Autodesk Fusion 360 part; units mm, degrees
(part 6 of 8)
  line L127 (16.3165, -98.3227) -> (16.3216, -98.4252)
  spline S1733 degree 3 poles (16.3216, -98.4252) (16.3211, -98.483) (16.3393, -98.5285) (16.3548, -98.5317) knots 0 0 0 0 1 1 1 1
  spline S1734 degree 3 poles (16.3548, -98.5317) (16.3752, -98.5342) (16.3906, -98.8238) (16.3886, -99.1759) knots 0 0 0 0 1 1 1 1
  spline S1735 degree 3 poles (16.3886, -99.1759) (16.3893, -99.7137) (16.3719, -99.8792) (16.278, -100.2401) knots 0 0 0 0 1 1 1 1
  spline S1736 degree 3 poles (16.278, -100.2401) (16.2147, -100.4816) (16.1437, -100.6813) (16.1109, -100.7004) knots 0 0 0 0 1 1 1 1
  spline S1737 degree 3 poles (16.1109, -100.7004) (16.0808, -100.7217) (16.069, -100.7483) (16.0801, -100.7569) knots 0 0 0 0 1 1 1 1
  spline S1738 degree 3 poles (16.0801, -100.7569) (16.094, -100.7678) (15.9885, -100.8913) (15.8475, -101.0318) knots 0 0 0 0 1 1 1 1
  spline S1739 degree 3 poles (15.8475, -101.0318) (15.7042, -101.1751) (15.5774, -101.3088) (15.5594, -101.326) knots 0 0 0 0 1 1 1 1
  spline S1740 degree 3 poles (15.5594, -101.326) (15.5442, -101.3455) (15.5244, -101.3479) (15.5198, -101.3309) knots 0 0 0 0 1 1 1 1
  spline S1741 degree 3 poles (15.5198, -101.3309) (15.5124, -101.3117) (15.4904, -101.3169) (15.473, -101.3392) knots 0 0 0 0 1 1 1 1
  spline S1742 degree 3 poles (15.473, -101.3392) (15.4448, -101.3753) (15.4503, -101.3796) (15.5098, -101.3724) knots 0 0 0 0 1 1 1 1
  spline S1743 degree 3 poles (15.5098, -101.3724) (15.5472, -101.3703) (15.7087, -101.2323) (15.8901, -101.0517) knots 0 0 0 0 1 1 1 1
  line L128 (15.8901, -101.0517) -> (16.2039, -100.7417)
  line L129 (16.2039, -100.7417) -> (16.3228, -100.2974)
  spline S1744 degree 3 poles (16.3228, -100.2974) (16.4479, -99.8221) (16.4656, -99.7822) (16.538, -99.7985) knots 0 0 0 0 1 1 1 1
  spline S1745 degree 3 poles (16.538, -99.7985) (16.5618, -99.8081) (16.555, -99.7939) (16.5195, -99.7706) knots 0 0 0 0 1 1 1 1
  spline S1746 degree 3 poles (16.5195, -99.7706) (16.454, -99.7284) (16.4546, -99.6931) (16.4526, -96.2577) knots 0 0 0 0 1 1 1 1
  spline S1747 degree 3 poles (16.4526, -96.2577) (16.4536, -95.6318) (16.4543, -95.0235) (16.4558, -94.9128) knots 0 0 0 0 1 1 1 1
  spline S1748 degree 3 poles (16.4558, -94.9128) (16.4567, -94.797) (16.4542, -94.2042) (16.4543, -93.591) knots 0 0 0 0 1 1 1 1
  spline S1749 degree 3 poles (16.4543, -93.591) (16.4524, -89.2558) (16.4467, -89.7215) (16.5046, -89.7219) knots 0 0 0 0 1 1 1 1
  spline S1750 degree 3 poles (16.5046, -89.7219) (16.525, -89.7245) (16.6036, -89.7098) (16.6773, -89.6957) knots 0 0 0 0 1 1 1 1
  spline S1751 degree 3 poles (16.6773, -89.6957) (16.7998, -89.6706) (16.7971, -89.6684) (16.6352, -89.6808) knots 0 0 0 0 1 1 1 1
  line L130 (16.6352, -89.6808) -> (16.4585, -89.6949)
  line L131 (16.4585, -89.6949) -> (16.4072, -89.5429)
  spline S1752 degree 3 poles (16.4072, -89.5429) (16.3814, -89.4556) (16.3356, -89.3079) (16.308, -89.2057) knots 0 0 0 0 1 1 1 1
  spline S1753 degree 3 poles (16.308, -89.2057) (16.281, -89.1085) (16.2542, -89.0339) (16.2455, -89.045) knots 0 0 0 0 1 1 1 1
  spline S1754 degree 3 poles (16.2455, -89.045) (16.2368, -89.0561) (16.2298, -89.0193) (16.2274, -88.9593) knots 0 0 0 0 1 1 1 1
  line L132 (16.2274, -88.9593) -> (16.2274, -88.8562)
  line L133 (16.2274, -88.8562) -> (16.1628, -88.9446)
  spline S1755 degree 3 poles (16.1628, -88.9446) (16.1222, -89.0023) (16.1096, -89.0642) (16.1256, -89.1125) knots 0 0 0 0 1 1 1 1
  spline S1756 degree 3 poles (16.3207, -89.3499) (16.3449, -89.445) (16.358, -89.5313) (16.3515, -89.5397) knots 0 0 0 0 1 1 1 1
  spline S1757 degree 3 poles (16.3515, -89.5397) (16.3471, -89.5452) (16.3232, -89.4728) (16.2989, -89.3777) knots 0 0 0 0 1 1 1 1
  spline S1758 degree 3 poles (16.2989, -89.3777) (16.2747, -89.2827) (16.2616, -89.1963) (16.2681, -89.188) knots 0 0 0 0 1 1 1 1
  spline S1759 degree 3 poles (16.2681, -89.188) (16.2724, -89.1824) (16.2964, -89.2549) (16.3207, -89.3499) knots 0 0 0 0 1 1 1 1
  spline S1760 degree 3 poles (16.3839, -89.5784) (16.3895, -89.5828) (16.3943, -89.6224) (16.3942, -89.6626) knots 0 0 0 0 1 1 1 1
  spline S1761 degree 3 poles (16.3942, -89.6626) (16.3956, -89.7353) (16.3907, -89.7359) (16.3744, -89.665) knots 0 0 0 0 1 1 1 1
  spline S1762 degree 3 poles (16.3744, -89.665) (16.3582, -89.5941) (16.3617, -89.561) (16.3839, -89.5784) knots 0 0 0 0 1 1 1 1
  spline S1763 degree 3 poles (16.3869, -97.9748) (16.3958, -98.0265) (16.3926, -98.0822) (16.3795, -98.0989) knots 0 0 0 0 1 1 1 1
  spline S1764 degree 3 poles (16.3795, -98.0989) (16.3637, -98.1134) (16.3517, -98.0771) (16.3522, -98.0193) knots 0 0 0 0 1 1 1 1
  spline S1765 degree 3 poles (16.3522, -98.0193) (16.3451, -97.8794) (16.3646, -97.8544) (16.3869, -97.9748) knots 0 0 0 0 1 1 1 1
  spline S1766 degree 3 poles (6.4751, -101.6422) (6.4707, -101.688) (6.4876, -101.7236) (6.5074, -101.7212) knots 0 0 0 0 1 1 1 1
  spline S1767 degree 3 poles (6.5074, -101.7212) (6.5272, -101.7188) (6.5375, -101.6999) (6.5295, -101.6758) knots 0 0 0 0 1 1 1 1
  spline S1768 degree 3 poles (6.5295, -101.6758) (6.5215, -101.6516) (6.5238, -101.6086) (6.5328, -101.5799) knots 0 0 0 0 1 1 1 1
  spline S1769 degree 3 poles (6.5328, -101.5799) (6.5424, -101.5561) (6.535, -101.5369) (6.5137, -101.547) knots 0 0 0 0 1 1 1 1
  spline S1770 degree 3 poles (6.5137, -101.547) (6.4917, -101.5522) (6.4746, -101.5971) (6.4751, -101.6422) knots 0 0 0 0 1 1 1 1
  spline S1771 degree 3 poles (16.7866, -88.5186) (16.8252, -88.5667) (16.8384, -88.5726) (16.8336, -88.533) knots 0 0 0 0 1 1 1 1
  spline S1772 degree 3 poles (16.8336, -88.533) (16.8305, -88.5082) (16.8065, -88.476) (16.7827, -88.4663) knots 0 0 0 0 1 1 1 1
  spline S1773 degree 3 poles (16.7827, -88.4663) (16.7539, -88.4573) (16.7591, -88.4793) (16.7866, -88.5186) knots 0 0 0 0 1 1 1 1
  spline S1774 degree 3 poles (6.7487, -102.0083) (6.7647, -102.0566) (6.7792, -102.0724) (6.7833, -102.0442) knots 0 0 0 0 1 1 1 1
  spline S1775 degree 3 poles (6.7833, -102.0442) (6.7852, -102.0189) (6.8218, -101.9892) (6.8636, -101.9816) knots 0 0 0 0 1 1 1 1
  spline S1776 degree 3 poles (6.8636, -101.9816) (6.9268, -101.9638) (6.9268, -101.9638) (6.8711, -101.9606) knots 0 0 0 0 1 1 1 1
  spline S1777 degree 3 poles (6.8711, -101.9606) (6.8358, -101.9599) (6.7845, -101.9511) (6.7606, -101.9414) knots 0 0 0 0 1 1 1 1
  spline S1778 degree 3 poles (6.7606, -101.9414) (6.7319, -101.9324) (6.7272, -101.9556) (6.7487, -102.0083) knots 0 0 0 0 1 1 1 1
  spline S1779 degree 3 poles (8.4157, -99.7829) (8.4296, -99.7938) (8.4739, -99.8059) (8.507, -99.8094) knots 0 0 0 0 1 1 1 1
  spline S1780 degree 3 poles (8.507, -99.8094) (8.5401, -99.8129) (8.5565, -99.8033) (8.5426, -99.7925) knots 0 0 0 0 1 1 1 1
  spline S1781 degree 3 poles (8.5426, -99.7925) (8.5259, -99.7794) (8.4845, -99.7695) (8.4514, -99.766) knots 0 0 0 0 1 1 1 1
  spline S1782 degree 3 poles (8.4514, -99.766) (8.4183, -99.7625) (8.3991, -99.7699) (8.4157, -99.7829) knots 0 0 0 0 1 1 1 1
  spline S1783 degree 3 poles (16.9973, -89.2116) (17.0136, -89.2824) (17.0185, -89.2818) (17.0171, -89.2091) knots 0 0 0 0 1 1 1 1
  spline S1784 degree 3 poles (17.0171, -89.2091) (17.0172, -89.1689) (17.0124, -89.1293) (17.0068, -89.1249) knots 0 0 0 0 1 1 1 1
  spline S1785 degree 3 poles (17.0068, -89.1249) (16.9846, -89.1076) (16.9811, -89.1407) (16.9973, -89.2116) knots 0 0 0 0 1 1 1 1
  spline S1786 degree 3 poles (8.7033, -99.8733) (8.7172, -99.8841) (8.7614, -99.8963) (8.7945, -99.8998) knots 0 0 0 0 1 1 1 1
  spline S1787 degree 3 poles (8.7945, -99.8998) (8.8276, -99.9032) (8.844, -99.8937) (8.8301, -99.8828) knots 0 0 0 0 1 1 1 1
  spline S1788 degree 3 poles (8.8301, -99.8828) (8.8134, -99.8698) (8.772, -99.8598) (8.7389, -99.8563) knots 0 0 0 0 1 1 1 1
  spline S1789 degree 3 poles (8.7389, -99.8563) (8.7058, -99.8529) (8.6866, -99.8602) (8.7033, -99.8733) knots 0 0 0 0 1 1 1 1
  spline S1790 degree 3 poles (11.2338, -96.6572) (11.2477, -96.6681) (11.2824, -96.6638) (11.3103, -96.6453) knots 0 0 0 0 1 1 1 1
  spline S1791 degree 3 poles (11.3103, -96.6453) (11.3546, -96.6173) (11.354, -96.6123) (11.294, -96.6147) knots 0 0 0 0 1 1 1 1
  spline S1792 degree 3 poles (11.294, -96.6147) (11.2163, -96.6167) (11.1977, -96.629) (11.2338, -96.6572) knots 0 0 0 0 1 1 1 1
  spline S1793 degree 3 poles (17.0434, -89.3818) (17.0596, -89.4527) (17.0646, -89.4521) (17.0632, -89.3794) knots 0 0 0 0 1 1 1 1
  spline S1794 degree 3 poles (17.0632, -89.3794) (17.0633, -89.3392) (17.0584, -89.2996) (17.0528, -89.2952) knots 0 0 0 0 1 1 1 1
  spline S1795 degree 3 poles (17.0528, -89.2952) (17.0306, -89.2778) (17.0271, -89.3109) (17.0434, -89.3818) knots 0 0 0 0 1 1 1 1
  spline S1796 degree 3 poles (15.3767, -91.5895) (15.3841, -91.6087) (15.4023, -91.614) (15.4132, -91.6001) knots 0 0 0 0 1 1 1 1
  spline S1797 degree 3 poles (15.4132, -91.6001) (15.4262, -91.5834) (15.4232, -91.5587) (15.4093, -91.5478) knots 0 0 0 0 1 1 1 1
  spline S1798 degree 3 poles (15.4093, -91.5478) (15.3926, -91.5348) (15.3772, -91.5317) (15.3728, -91.5372) knots 0 0 0 0 1 1 1 1
  spline S1799 degree 3 poles (15.3728, -91.5372) (15.3663, -91.5456) (15.3666, -91.5682) (15.3767, -91.5895) knots 0 0 0 0 1 1 1 1
  spline S1800 degree 3 poles (17.0851, -89.5577) (17.0917, -89.6121) (17.0843, -89.6332) (17.062, -89.6158) knots 0 0 0 0 1 1 1 1
  spline S1801 degree 3 poles (17.062, -89.6158) (17.0426, -89.6006) (17.0178, -89.6036) (17.0026, -89.6231) knots 0 0 0 0 1 1 1 1
  spline S1802 degree 3 poles (17.0026, -89.6231) (16.9831, -89.6481) (16.9914, -89.6546) (17.036, -89.6491) knots 0 0 0 0 1 1 1 1
  spline S1803 degree 3 poles (17.036, -89.6491) (17.0805, -89.6437) (17.0978, -89.6617) (17.1141, -89.7325) knots 0 0 0 0 1 1 1 1
  spline S1804 degree 3 poles (17.1141, -89.7325) (17.1257, -89.7864) (17.1258, -89.7462) (17.1214, -89.6487) knots 0 0 0 0 1 1 1 1
  spline S1805 degree 3 poles (17.1214, -89.6487) (17.112, -89.5518) (17.1017, -89.4677) (17.0961, -89.4633) knots 0 0 0 0 1 1 1 1
  spline S1806 degree 3 poles (17.0961, -89.4633) (17.0794, -89.4503) (17.0775, -89.4757) (17.0851, -89.5577) knots 0 0 0 0 1 1 1 1
  spline S1807 degree 3 poles (9.0301, -99.9764) (9.0616, -99.9876) (9.099, -100.0257) (9.1088, -100.0648) knots 0 0 0 0 1 1 1 1
  spline S1808 degree 3 poles (9.1088, -100.0648) (9.1232, -100.1208) (9.126, -100.123) (9.1221, -100.0707) knots 0 0 0 0 1 1 1 1
  spline S1809 degree 3 poles (9.1221, -100.0707) (9.121, -100.0205) (9.1498, -99.9893) (9.2638, -99.9351) knots 0 0 0 0 1 1 1 1
  spline S1810 degree 3 poles (9.2638, -99.9351) (9.3416, -99.8929) (9.3722, -99.8766) (9.3289, -99.892) knots 0 0 0 0 1 1 1 1
  spline S1811 degree 3 poles (9.3289, -99.892) (9.2877, -99.9046) (9.1871, -99.9245) (9.1106, -99.9364) knots 0 0 0 0 1 1 1 1
  spline S1812 degree 3 poles (9.1106, -99.9364) (9.0243, -99.9495) (8.9936, -99.9658) (9.0301, -99.9764) knots 0 0 0 0 1 1 1 1
  spline S1813 degree 3 poles (11.9407, -96.5604) (12.1041, -96.5403) (12.2422, -96.5184) (12.2465, -96.5128) knots 0 0 0 0 1 1 1 1
  spline S1814 degree 3 poles (12.2465, -96.5128) (12.253, -96.5045) (12.1259, -96.5125) (11.9625, -96.5326) knots 0 0 0 0 1 1 1 1
  spline S1815 degree 3 poles (11.9625, -96.5326) (11.799, -96.5527) (11.661, -96.5746) (11.6567, -96.5802) knots 0 0 0 0 1 1 1 1
  spline S1816 degree 3 poles (11.6567, -96.5802) (11.6501, -96.5885) (11.7773, -96.5805) (11.9407, -96.5604) knots 0 0 0 0 1 1 1 1
  line L134 (17.1133, -89.9513) -> (17.136, -90.0541)
  line L135 (17.136, -90.0541) -> (17.1331, -89.9489)
  spline S1817 degree 3 poles (17.1331, -89.9489) (17.1287, -89.8514) (17.1195, -89.8173) (17.1021, -89.8396) knots 0 0 0 0 1 1 1 1
  spline S1818 degree 3 poles (17.1021, -89.8396) (17.0977, -89.8451) (17.1038, -89.8947) (17.1133, -89.9513) knots 0 0 0 0 1 1 1 1
  spline S1819 degree 3 poles (7.9987, -101.606) (8.0126, -101.6168) (8.0374, -101.6138) (8.0504, -101.5971) knots 0 0 0 0 1 1 1 1
  spline S1820 degree 3 poles (8.0504, -101.5971) (8.0613, -101.5832) (8.0517, -101.5668) (8.0313, -101.5643) knots 0 0 0 0 1 1 1 1
  spline S1821 degree 3 poles (8.0313, -101.5643) (8.0081, -101.5596) (7.9861, -101.5648) (7.9796, -101.5731) knots 0 0 0 0 1 1 1 1
  spline S1822 degree 3 poles (7.9796, -101.5731) (7.9752, -101.5787) (7.982, -101.5929) (7.9987, -101.606) knots 0 0 0 0 1 1 1 1
  spline S1823 degree 3 poles (7.3497, -102.6658) (7.4478, -102.6663) (7.5348, -102.6582) (7.5413, -102.6498) knots 0 0 0 0 1 1 1 1
  spline S1824 degree 3 poles (7.5413, -102.6498) (7.5456, -102.6443) (7.4695, -102.6385) (7.3714, -102.638) knots 0 0 0 0 1 1 1 1
  spline S1825 degree 3 poles (7.3714, -102.638) (7.2734, -102.6375) (7.1864, -102.6457) (7.1799, -102.654) knots 0 0 0 0 1 1 1 1
  spline S1826 degree 3 poles (7.1799, -102.654) (7.1755, -102.6596) (7.2516, -102.6653) (7.3497, -102.6658) knots 0 0 0 0 1 1 1 1
  line L136 (9.1141, -100.333) -> (9.1398, -100.4606)
  line L137 (9.1398, -100.4606) -> (9.1339, -100.3306)
  spline S1827 degree 3 poles (9.1339, -100.3306) (9.1276, -100.2585) (9.1203, -100.1991) (9.1147, -100.1947) knots 0 0 0 0 1 1 1 1
  spline S1828 degree 3 poles (9.1147, -100.1947) (9.0925, -100.1773) (9.0946, -100.2148) (9.1141, -100.333) knots 0 0 0 0 1 1 1 1
  spline S1829 degree 3 poles (9.4989, -99.8233) (9.5072, -99.8299) (9.5462, -99.82) (9.5868, -99.8025) knots 0 0 0 0 1 1 1 1
  spline S1830 degree 3 poles (9.5868, -99.8025) (9.6274, -99.7849) (9.6525, -99.7643) (9.6469, -99.7599) knots 0 0 0 0 1 1 1 1
  spline S1831 degree 3 poles (9.6469, -99.7599) (9.6386, -99.7534) (9.5996, -99.7632) (9.559, -99.7808) knots 0 0 0 0 1 1 1 1
  spline S1832 degree 3 poles (9.559, -99.7808) (9.5184, -99.7983) (9.4933, -99.819) (9.4989, -99.8233) knots 0 0 0 0 1 1 1 1
  spline S1833 degree 3 poles (17.1128, -90.1524) (17.1291, -90.2233) (17.134, -90.2227) (17.1327, -90.15) knots 0 0 0 0 1 1 1 1
  spline S1834 degree 3 poles (17.1327, -90.15) (17.1327, -90.1098) (17.1279, -90.0701) (17.1223, -90.0658) knots 0 0 0 0 1 1 1 1
  spline S1835 degree 3 poles (17.1223, -90.0658) (17.1001, -90.0484) (17.0966, -90.0815) (17.1128, -90.1524) knots 0 0 0 0 1 1 1 1
  line L138 (9.1228, -100.6084) -> (9.1485, -100.7359)
  line L139 (9.1485, -100.7359) -> (9.1426, -100.606)
  spline S1836 degree 3 poles (9.1426, -100.606) (9.1363, -100.5339) (9.129, -100.4745) (9.1234, -100.4701) knots 0 0 0 0 1 1 1 1
  spline S1837 degree 3 poles (9.1234, -100.4701) (9.1012, -100.4527) (9.1032, -100.4902) (9.1228, -100.6084) knots 0 0 0 0 1 1 1 1
  line L140 (17.1124, -90.3535) -> (17.1351, -90.4563)
  line L141 (17.1351, -90.4563) -> (17.1322, -90.3511)
  spline S1838 degree 3 poles (17.1322, -90.3511) (17.1278, -90.2536) (17.1186, -90.2196) (17.1012, -90.2418) knots 0 0 0 0 1 1 1 1
  spline S1839 degree 3 poles (17.1012, -90.2418) (17.0969, -90.2474) (17.1029, -90.2969) (17.1124, -90.3535) knots 0 0 0 0 1 1 1 1
  spline S1840 degree 3 poles (7.752, -102.6667) (7.85, -102.6672) (7.937, -102.6591) (7.9435, -102.6507) knots 0 0 0 0 1 1 1 1
  spline S1841 degree 3 poles (7.9435, -102.6507) (7.9479, -102.6452) (7.8718, -102.6394) (7.7737, -102.6389) knots 0 0 0 0 1 1 1 1
  spline S1842 degree 3 poles (7.7737, -102.6389) (7.6756, -102.6384) (7.5886, -102.6465) (7.5821, -102.6549) knots 0 0 0 0 1 1 1 1
  spline S1843 degree 3 poles (7.5821, -102.6549) (7.5778, -102.6604) (7.6539, -102.6662) (7.752, -102.6667) knots 0 0 0 0 1 1 1 1
  spline S1844 degree 3 poles (17.112, -90.5546) (17.1282, -90.6255) (17.1332, -90.6249) (17.1318, -90.5522) knots 0 0 0 0 1 1 1 1
  spline S1845 degree 3 poles (17.1318, -90.5522) (17.1304, -90.4795) (17.119, -90.4482) (17.1016, -90.4705) knots 0 0 0 0 1 1 1 1
  spline S1846 degree 3 poles (17.1016, -90.4705) (17.0973, -90.476) (17.1022, -90.5156) (17.112, -90.5546) knots 0 0 0 0 1 1 1 1
  spline S1847 degree 3 poles (7.2792, -103.2374) (7.2847, -103.2418) (7.3243, -103.2369) (7.3655, -103.2243) knots 0 0 0 0 1 1 1 1
  spline S1848 degree 3 poles (7.3655, -103.2243) (7.4342, -103.2109) (7.4336, -103.2059) (7.3609, -103.2073) knots 0 0 0 0 1 1 1 1
  spline S1849 degree 3 poles (7.3609, -103.2073) (7.2882, -103.2087) (7.2569, -103.2201) (7.2792, -103.2374) knots 0 0 0 0 1 1 1 1
  line L142 (17.1115, -90.7557) -> (17.1342, -90.8585)
  line L143 (17.1342, -90.8585) -> (17.1313, -90.7533)
  spline S1850 degree 3 poles (17.1313, -90.7533) (17.1269, -90.6558) (17.1177, -90.6218) (17.1003, -90.644) knots 0 0 0 0 1 1 1 1
  spline S1851 degree 3 poles (17.1003, -90.644) (17.096, -90.6496) (17.1021, -90.6991) (17.1115, -90.7557) knots 0 0 0 0 1 1 1 1
  spline S1852 degree 3 poles (13.8781, -94.9402) (13.8854, -94.9594) (13.9037, -94.9647) (13.9145, -94.9508) knots 0 0 0 0 1 1 1 1
  spline S1853 degree 3 poles (13.9145, -94.9508) (13.9276, -94.9342) (13.9245, -94.9094) (13.9106, -94.8985) knots 0 0 0 0 1 1 1 1
  spline S1854 degree 3 poles (13.9106, -94.8985) (13.894, -94.8855) (13.8785, -94.8824) (13.8742, -94.8879) knots 0 0 0 0 1 1 1 1
  spline S1855 degree 3 poles (13.8742, -94.8879) (13.8676, -94.8963) (13.8679, -94.9189) (13.8781, -94.9402) knots 0 0 0 0 1 1 1 1
  spline S1856 degree 3 poles (8.7645, -101.5999) (8.7849, -101.6024) (8.8097, -101.5994) (8.8162, -101.591) knots 0 0 0 0 1 1 1 1
  spline S1857 degree 3 poles (8.8162, -101.591) (8.8205, -101.5855) (8.811, -101.5691) (8.7971, -101.5582) knots 0 0 0 0 1 1 1 1
  spline S1858 degree 3 poles (8.7971, -101.5582) (8.7804, -101.5452) (8.7584, -101.5504) (8.7454, -101.5671) knots 0 0 0 0 1 1 1 1
  spline S1859 degree 3 poles (8.7454, -101.5671) (8.7345, -101.581) (8.7413, -101.5952) (8.7645, -101.5999) knots 0 0 0 0 1 1 1 1
  spline S1860 degree 3 poles (17.1111, -90.9569) (17.1273, -91.0278) (17.1323, -91.0271) (17.1309, -90.9544) knots 0 0 0 0 1 1 1 1
  spline S1861 degree 3 poles (17.1309, -90.9544) (17.131, -90.9142) (17.1261, -90.8746) (17.1206, -90.8702) knots 0 0 0 0 1 1 1 1
  spline S1862 degree 3 poles (17.1206, -90.8702) (17.0983, -90.8529) (17.0948, -90.886) (17.1111, -90.9569) knots 0 0 0 0 1 1 1 1
  spline S1863 degree 3 poles (13.0195, -96.2168) (13.0334, -96.2277) (13.0498, -96.2181) (13.0523, -96.1977) knots 0 0 0 0 1 1 1 1
  spline S1864 degree 3 poles (13.0523, -96.1977) (13.057, -96.1745) (13.0518, -96.1525) (13.0434, -96.146) knots 0 0 0 0 1 1 1 1
  spline S1865 degree 3 poles (13.0434, -96.146) (13.0379, -96.1417) (13.0236, -96.1485) (13.0106, -96.1651) knots 0 0 0 0 1 1 1 1
  spline S1866 degree 3 poles (13.0106, -96.1651) (12.9997, -96.179) (13.0028, -96.2038) (13.0195, -96.2168) knots 0 0 0 0 1 1 1 1
  spline S1867 degree 3 poles (8.1542, -102.6676) (8.2523, -102.6681) (8.3392, -102.6599) (8.3457, -102.6516) knots 0 0 0 0 1 1 1 1
  spline S1868 degree 3 poles (8.3457, -102.6516) (8.3501, -102.646) (8.274, -102.6403) (8.1759, -102.6398) knots 0 0 0 0 1 1 1 1
  spline S1869 degree 3 poles (8.1759, -102.6398) (8.0778, -102.6392) (7.9909, -102.6474) (7.9843, -102.6558) knots 0 0 0 0 1 1 1 1
  spline S1870 degree 3 poles (7.9843, -102.6558) (7.98, -102.6613) (8.0561, -102.667) (8.1542, -102.6676) knots 0 0 0 0 1 1 1 1
  line L144 (17.1106, -91.158) -> (17.1333, -91.2607)
  line L145 (17.1333, -91.2607) -> (17.1305, -91.1555)
  spline S1871 degree 3 poles (17.1305, -91.1555) (17.126, -91.0581) (17.1168, -91.024) (17.0994, -91.0463) knots 0 0 0 0 1 1 1 1
  spline S1872 degree 3 poles (17.0994, -91.0463) (17.0951, -91.0518) (17.1012, -91.1013) (17.1106, -91.158) knots 0 0 0 0 1 1 1 1
  spline S1873 degree 3 poles (16.7444, -91.6955) (16.7499, -91.6999) (16.7896, -91.695) (16.8307, -91.6824) knots 0 0 0 0 1 1 1 1
  spline S1874 degree 3 poles (16.8307, -91.6824) (16.8994, -91.669) (16.8988, -91.664) (16.8261, -91.6654) knots 0 0 0 0 1 1 1 1
  spline S1875 degree 3 poles (16.8261, -91.6654) (16.7534, -91.6668) (16.7221, -91.6782) (16.7444, -91.6955) knots 0 0 0 0 1 1 1 1
  spline S1876 degree 3 poles (9.0702, -101.5925) (9.1119, -101.6251) (9.2143, -101.6201) (9.2129, -101.5876) knots 0 0 0 0 1 1 1 1
  spline S1877 degree 3 poles (9.2129, -101.5876) (9.2083, -101.5705) (9.1718, -101.5599) (9.1272, -101.5654) knots 0 0 0 0 1 1 1 1
  spline S1878 degree 3 poles (9.1272, -101.5654) (9.0826, -101.5709) (9.0563, -101.5817) (9.0702, -101.5925) knots 0 0 0 0 1 1 1 1
  spline S1879 degree 3 poles (17.1031, -91.5057) (17.1096, -91.7839) (17.1239, -91.8802) (17.1302, -91.706) knots 0 0 0 0 1 1 1 1
  spline S1880 degree 3 poles (17.1302, -91.706) (17.141, -91.5488) (17.1265, -91.2465) (17.1113, -91.266) knots 0 0 0 0 1 1 1 1
  spline S1881 degree 3 poles (17.1113, -91.266) (17.1048, -91.2743) (17.1027, -91.3801) (17.1031, -91.5057) knots 0 0 0 0 1 1 1 1
  spline S1882 degree 3 poles (9.1018, -101.7068) (9.1074, -101.7111) (9.147, -101.7062) (9.1882, -101.6936) knots 0 0 0 0 1 1 1 1
  spline S1883 degree 3 poles (9.1882, -101.6936) (9.2569, -101.6802) (9.2563, -101.6752) (9.1836, -101.6766) knots 0 0 0 0 1 1 1 1
  spline S1884 degree 3 poles (9.1836, -101.6766) (9.1109, -101.678) (9.0796, -101.6894) (9.1018, -101.7068) knots 0 0 0 0 1 1 1 1
  spline S1885 degree 3 poles (16.918, -91.6969) (16.9235, -91.7012) (16.9588, -91.7019) (16.9928, -91.6927) knots 0 0 0 0 1 1 1 1
  spline S1886 degree 3 poles (16.9928, -91.6927) (17.0417, -91.6817) (17.0526, -91.6678) (17.0378, -91.6294) knots 0 0 0 0 1 1 1 1
  spline S1887 degree 3 poles (17.0378, -91.6294) (17.0271, -91.603) (17.0187, -91.5965) (17.019, -91.6191) knots 0 0 0 0 1 1 1 1
  spline S1888 degree 3 poles (17.019, -91.6191) (17.0214, -91.6389) (16.9969, -91.6645) (16.9629, -91.6737) knots 0 0 0 0 1 1 1 1
  spline S1889 degree 3 poles (16.9629, -91.6737) (16.931, -91.6802) (16.9096, -91.6903) (16.918, -91.6969) knots 0 0 0 0 1 1 1 1
  spline S1890 degree 3 poles (7.4573, -103.869) (7.4628, -103.8734) (7.5024, -103.8685) (7.5436, -103.8559) knots 0 0 0 0 1 1 1 1
  spline S1891 degree 3 poles (7.5436, -103.8559) (7.6123, -103.8424) (7.6117, -103.8375) (7.539, -103.8389) knots 0 0 0 0 1 1 1 1
  spline S1892 degree 3 poles (7.539, -103.8389) (7.4663, -103.8403) (7.435, -103.8517) (7.4573, -103.869) knots 0 0 0 0 1 1 1 1
  spline S1893 degree 3 poles (8.3912, -102.6737) (8.3967, -102.678) (8.4364, -102.6731) (8.4775, -102.6605) knots 0 0 0 0 1 1 1 1
  spline S1894 degree 3 poles (8.4775, -102.6605) (8.5462, -102.6471) (8.5456, -102.6421) (8.4729, -102.6435) knots 0 0 0 0 1 1 1 1
  spline S1895 degree 3 poles (8.4729, -102.6435) (8.4002, -102.6449) (8.3689, -102.6563) (8.3912, -102.6737) knots 0 0 0 0 1 1 1 1
  spline S1896 degree 3 poles (9.4035, -101.5843) (9.4174, -101.5951) (9.4421, -101.5921) (9.4551, -101.5754) knots 0 0 0 0 1 1 1 1
  spline S1897 degree 3 poles (9.4551, -101.5754) (9.466, -101.5615) (9.4565, -101.5451) (9.436, -101.5426) knots 0 0 0 0 1 1 1 1
  spline S1898 degree 3 poles (9.436, -101.5426) (9.4128, -101.5379) (9.3909, -101.5431) (9.3843, -101.5514) knots 0 0 0 0 1 1 1 1
  spline S1899 degree 3 poles (9.3843, -101.5514) (9.38, -101.557) (9.3868, -101.5712) (9.4035, -101.5843) knots 0 0 0 0 1 1 1 1
  spline S1900 degree 3 poles (9.3277, -101.7042) (9.3333, -101.7085) (9.3729, -101.7036) (9.4141, -101.691) knots 0 0 0 0 1 1 1 1
  spline S1901 degree 3 poles (9.4141, -101.691) (9.4828, -101.6776) (9.4822, -101.6726) (9.4095, -101.674) knots 0 0 0 0 1 1 1 1
  spline S1902 degree 3 poles (9.4095, -101.674) (9.3367, -101.6754) (9.3055, -101.6868) (9.3277, -101.7042) knots 0 0 0 0 1 1 1 1
  spline S1903 degree 3 poles (7.6831, -103.8664) (7.6887, -103.8708) (7.7283, -103.8659) (7.7695, -103.8533) knots 0 0 0 0 1 1 1 1
  spline S1904 degree 3 poles (7.7695, -103.8533) (7.8382, -103.8398) (7.8376, -103.8349) (7.7649, -103.8363) knots 0 0 0 0 1 1 1 1
  spline S1905 degree 3 poles (7.7649, -103.8363) (7.6922, -103.8377) (7.6609, -103.849) (7.6831, -103.8664) knots 0 0 0 0 1 1 1 1
  spline S1906 degree 3 poles (10.874, -99.9083) (10.9046, -99.9322) (10.9195, -99.9304) (10.9037, -99.9047) knots 0 0 0 0 1 1 1 1
  spline S1907 degree 3 poles (10.9037, -99.9047) (10.8908, -99.8811) (10.8636, -99.8644) (10.8487, -99.8662) knots 0 0 0 0 1 1 1 1
  spline S1908 degree 3 poles (10.8487, -99.8662) (10.8311, -99.8658) (10.8413, -99.8872) (10.874, -99.9083) knots 0 0 0 0 1 1 1 1
  line L146 (17.1089, -91.9624) -> (17.1316, -92.0652)
  line L147 (17.1316, -92.0652) -> (17.1287, -91.96)
  spline S1909 degree 3 poles (17.1287, -91.96) (17.1242, -91.9027) (17.1181, -91.8532) (17.1125, -91.8489) knots 0 0 0 0 1 1 1 1
  spline S1910 degree 3 poles (17.1125, -91.8489) (17.0903, -91.8315) (17.0896, -91.8668) (17.1089, -91.9624) knots 0 0 0 0 1 1 1 1
  spline S1911 degree 3 poles (7.717, -103.9377) (7.7226, -103.942) (7.7622, -103.9371) (7.8034, -103.9245) knots 0 0 0 0 1 1 1 1
  spline S1912 degree 3 poles (7.8034, -103.9245) (7.8721, -103.9111) (7.8715, -103.9061) (7.7988, -103.9075) knots 0 0 0 0 1 1 1 1
  spline S1913 degree 3 poles (7.7988, -103.9075) (7.726, -103.9089) (7.6948, -103.9203) (7.717, -103.9377) knots 0 0 0 0 1 1 1 1
  spline S1914 degree 3 poles (7.909, -103.8638) (7.9146, -103.8682) (7.9542, -103.8633) (7.9954, -103.8507) knots 0 0 0 0 1 1 1 1
  spline S1915 degree 3 poles (7.9954, -103.8507) (8.0641, -103.8372) (8.0635, -103.8323) (7.9907, -103.8337) knots 0 0 0 0 1 1 1 1
  spline S1916 degree 3 poles (7.9907, -103.8337) (7.918, -103.8351) (7.8868, -103.8464) (7.909, -103.8638) knots 0 0 0 0 1 1 1 1
  line L148 (17.1115, -92.1883) -> (17.1342, -92.2911)
  line L149 (17.1342, -92.2911) -> (17.1313, -92.1859)
  spline S1917 degree 3 poles (17.1313, -92.1859) (17.1269, -92.0884) (17.1177, -92.0543) (17.1003, -92.0766) knots 0 0 0 0 1 1 1 1
  spline S1918 degree 3 poles (17.1003, -92.0766) (17.0959, -92.0821) (17.102, -92.1317) (17.1115, -92.1883) knots 0 0 0 0 1 1 1 1
  spline S1919 degree 3 poles (11.087, -100.1285) (11.096, -100.2832) (11.0988, -100.2854) (11.1077, -100.1536) knots 0 0 0 0 1 1 1 1
  spline S1920 degree 3 poles (11.1077, -100.1536) (11.1113, -100.0803) (11.1232, -100.0135) (11.1319, -100.0023) knots 0 0 0 0 1 1 1 1
  spline S1921 degree 3 poles (11.1319, -100.0023) (11.1384, -99.994) (11.2272, -99.9605) (11.326, -99.9257) knots 0 0 0 0 1 1 1 1
  spline S1922 degree 3 poles (11.326, -99.9257) (11.5731, -99.8501) (11.5338, -99.8374) (11.2812, -99.9086) knots 0 0 0 0 1 1 1 1
  line L150 (11.2812, -99.9086) -> (11.0824, -99.9682)
  line L151 (11.0824, -99.9682) -> (11.087, -100.1285)
  spline S1923 degree 3 poles (9.0193, -102.6719) (9.0248, -102.6763) (9.0645, -102.6714) (9.1056, -102.6588) knots 0 0 0 0 1 1 1 1
  spline S1924 degree 3 poles (9.1056, -102.6588) (9.1743, -102.6454) (9.1737, -102.6404) (9.101, -102.6418) knots 0 0 0 0 1 1 1 1
  spline S1925 degree 3 poles (9.101, -102.6418) (9.0283, -102.6432) (8.997, -102.6546) (9.0193, -102.6719) knots 0 0 0 0 1 1 1 1
  spline S1926 degree 3 poles (9.3885, -102.1993) (9.3941, -102.2037) (9.4337, -102.1988) (9.4749, -102.1862) knots 0 0 0 0 1 1 1 1
  spline S1927 degree 3 poles (9.4749, -102.1862) (9.5436, -102.1728) (9.543, -102.1678) (9.4703, -102.1692) knots 0 0 0 0 1 1 1 1
  spline S1928 degree 3 poles (9.4703, -102.1692) (9.3975, -102.1706) (9.3663, -102.182) (9.3885, -102.1993) knots 0 0 0 0 1 1 1 1
  spline S1929 degree 3 poles (17.1111, -92.3894) (17.1273, -92.4603) (17.1323, -92.4597) (17.1309, -92.387) knots 0 0 0 0 1 1 1 1
  spline S1930 degree 3 poles (17.1309, -92.387) (17.131, -92.3468) (17.1261, -92.3071) (17.1205, -92.3028) knots 0 0 0 0 1 1 1 1
  spline S1931 degree 3 poles (17.1205, -92.3028) (17.0983, -92.2854) (17.0948, -92.3185) (17.1111, -92.3894) knots 0 0 0 0 1 1 1 1
  spline S1932 degree 3 poles (8.1192, -103.9385) (8.1248, -103.9429) (8.1644, -103.938) (8.2056, -103.9254) knots 0 0 0 0 1 1 1 1
  spline S1933 degree 3 poles (8.2056, -103.9254) (8.2743, -103.912) (8.2737, -103.907) (8.201, -103.9084) knots 0 0 0 0 1 1 1 1
  spline S1934 degree 3 poles (8.201, -103.9084) (8.1283, -103.9098) (8.097, -103.9212) (8.1192, -103.9385) knots 0 0 0 0 1 1 1 1
  line L152 (17.1106, -92.5905) -> (17.1333, -92.6933)
  line L153 (17.1333, -92.6933) -> (17.1304, -92.5881)
  spline S1935 degree 3 poles (17.1304, -92.5881) (17.126, -92.4906) (17.1168, -92.4566) (17.0994, -92.4788) knots 0 0 0 0 1 1 1 1
  spline S1936 degree 3 poles (17.0994, -92.4788) (17.0951, -92.4844) (17.1011, -92.5339) (17.1106, -92.5905) knots 0 0 0 0 1 1 1 1
  spline S1937 degree 3 poles (9.1956, -102.6754) (9.2012, -102.6798) (9.2359, -102.6755) (9.2727, -102.6685) knots 0 0 0 0 1 1 1 1
  spline S1938 degree 3 poles (9.2727, -102.6685) (9.3315, -102.6562) (9.3309, -102.6513) (9.2811, -102.6348) knots 0 0 0 0 1 1 1 1
  spline S1939 degree 3 poles (9.2811, -102.6348) (9.2313, -102.6183) (9.1651, -102.6515) (9.1956, -102.6754) knots 0 0 0 0 1 1 1 1
  spline S1940 degree 3 poles (10.0482, -101.5956) (10.0566, -101.6021) (10.0968, -101.6022) (10.1364, -101.5973) knots 0 0 0 0 1 1 1 1
  spline S1941 degree 3 poles (10.1364, -101.5973) (10.2184, -101.5898) (10.2144, -101.5777) (10.1282, -101.5506) knots 0 0 0 0 1 1 1 1
  spline S1942 degree 3 poles (10.1282, -101.5506) (10.0734, -101.5347) (10.0121, -101.5673) (10.0482, -101.5956) knots 0 0 0 0 1 1 1 1
  spline S1943 degree 3 poles (8.3048, -103.9761) (8.3156, -104.0024) (8.3239, -104.0089) (8.3236, -103.9863) knots 0 0 0 0 1 1 1 1
  spline S1944 degree 3 poles (8.3236, -103.9863) (8.3212, -103.9665) (8.3507, -103.9403) (8.3897, -103.9305) knots 0 0 0 0 1 1 1 1
  spline S1945 degree 3 poles (8.3897, -103.9305) (8.4507, -103.9154) (8.4479, -103.9133) (8.3773, -103.9119) knots 0 0 0 0 1 1 1 1
  spline S1946 degree 3 poles (8.3773, -103.9119) (8.287, -103.9129) (8.2799, -103.9163) (8.3048, -103.9761) knots 0 0 0 0 1 1 1 1
  spline S1947 degree 3 poles (11.5378, -99.8494) (11.5462, -99.856) (11.7548, -99.7952) (11.9991, -99.7174) knots 0 0 0 0 1 1 1 1
  spline S1948 degree 3 poles (11.9991, -99.7174) (12.2456, -99.6369) (12.4283, -99.5692) (12.4057, -99.5695) knots 0 0 0 0 1 1 1 1
  spline S1949 degree 3 poles (12.4057, -99.5695) (12.3571, -99.5629) (11.5211, -99.8364) (11.5378, -99.8494) knots 0 0 0 0 1 1 1 1
  line L154 (17.1132, -92.8164) -> (17.1359, -92.9192)
  line L155 (17.1359, -92.9192) -> (17.133, -92.814)
  spline S1950 degree 3 poles (17.133, -92.814) (17.1286, -92.7165) (17.1194, -92.6824) (17.102, -92.7047) knots 0 0 0 0 1 1 1 1
  spline S1951 degree 3 poles (17.102, -92.7047) (17.0977, -92.7102) (17.1038, -92.7598) (17.1132, -92.8164) knots 0 0 0 0 1 1 1 1
  spline S1952 degree 3 poles (8.379, -104.0072) (8.3845, -104.0115) (8.4242, -104.0067) (8.4653, -103.9941) knots 0 0 0 0 1 1 1 1
  spline S1953 degree 3 poles (8.4653, -103.9941) (8.5341, -103.9806) (8.5334, -103.9756) (8.4607, -103.977) knots 0 0 0 0 1 1 1 1
  spline S1954 degree 3 poles (8.4607, -103.977) (8.388, -103.9784) (8.3567, -103.9898) (8.379, -104.0072) knots 0 0 0 0 1 1 1 1
  spline S1955 degree 3 poles (9.7907, -102.2002) (9.7963, -102.2046) (9.8359, -102.1997) (9.8771, -102.1871) knots 0 0 0 0 1 1 1 1
  spline S1956 degree 3 poles (9.8771, -102.1871) (9.9458, -102.1736) (9.9452, -102.1687) (9.8725, -102.1701) knots 0 0 0 0 1 1 1 1
  spline S1957 degree 3 poles (9.8725, -102.1701) (9.7998, -102.1715) (9.7685, -102.1828) (9.7907, -102.2002) knots 0 0 0 0 1 1 1 1
  spline S1958 degree 3 poles (17.1128, -93.0175) (17.129, -93.0884) (17.134, -93.0878) (17.1326, -93.0151) knots 0 0 0 0 1 1 1 1
  spline S1959 degree 3 poles (17.1326, -93.0151) (17.1312, -92.9424) (17.1198, -92.9111) (17.1024, -92.9333) knots 0 0 0 0 1 1 1 1
  spline S1960 degree 3 poles (17.1024, -92.9333) (17.0981, -92.9389) (17.103, -92.9785) (17.1128, -93.0175) knots 0 0 0 0 1 1 1 1
  spline S1961 degree 3 poles (10.0089, -102.1961) (10.0491, -102.1961) (10.0924, -102.221) (10.1031, -102.2473) knots 0 0 0 0 1 1 1 1
  spline S1962 degree 3 poles (10.1031, -102.2473) (10.1179, -102.2857) (10.125, -102.2823) (10.1183, -102.2279) knots 0 0 0 0 1 1 1 1
  spline S1963 degree 3 poles (10.1183, -102.2279) (10.1144, -102.1756) (10.0984, -102.1675) (10.0219, -102.1794) knots 0 0 0 0 1 1 1 1
  spline S1964 degree 3 poles (10.0219, -102.1794) (9.9433, -102.1941) (9.9411, -102.1968) (10.0089, -102.1961) knots 0 0 0 0 1 1 1 1
  spline S1965 degree 3 poles (10.358, -101.7033) (10.3636, -101.7077) (10.4032, -101.7028) (10.4444, -101.6902) knots 0 0 0 0 1 1 1 1
  spline S1966 degree 3 poles (10.4444, -101.6902) (10.5131, -101.6767) (10.5125, -101.6718) (10.4398, -101.6732) knots 0 0 0 0 1 1 1 1
  spline S1967 degree 3 poles (10.4398, -101.6732) (10.3671, -101.6746) (10.3358, -101.6859) (10.358, -101.7033) knots 0 0 0 0 1 1 1 1
  spline S1968 degree 3 poles (8.6049, -104.0046) (8.6104, -104.0089) (8.65, -104.0041) (8.6912, -103.9915) knots 0 0 0 0 1 1 1 1
  spline S1969 degree 3 poles (8.6912, -103.9915) (8.7599, -103.978) (8.7593, -103.973) (8.6866, -103.9744) knots 0 0 0 0 1 1 1 1
  spline S1970 degree 3 poles (8.6866, -103.9744) (8.6139, -103.9758) (8.5826, -103.9872) (8.6049, -104.0046) knots 0 0 0 0 1 1 1 1
  line L156 (17.1123, -93.2186) -> (17.135, -93.3214)
  line L157 (17.135, -93.3214) -> (17.1321, -93.2162)
  spline S1971 degree 3 poles (17.1321, -93.2162) (17.1277, -93.1187) (17.1185, -93.0847) (17.1011, -93.1069) knots 0 0 0 0 1 1 1 1
  spline S1972 degree 3 poles (17.1011, -93.1069) (17.0968, -93.1125) (17.1029, -93.162) (17.1123, -93.2186) knots 0 0 0 0 1 1 1 1
  spline S1973 degree 3 poles (10.5993, -101.6008) (10.6197, -101.6033) (10.6445, -101.6003) (10.651, -101.5919) knots 0 0 0 0 1 1 1 1
  spline S1974 degree 3 poles (10.651, -101.5919) (10.6553, -101.5864) (10.6458, -101.57) (10.6319, -101.5591) knots 0 0 0 0 1 1 1 1
  spline S1975 degree 3 poles (10.6319, -101.5591) (10.6152, -101.5461) (10.5932, -101.5513) (10.5802, -101.568) knots 0 0 0 0 1 1 1 1
  spline S1976 degree 3 poles (10.5802, -101.568) (10.5693, -101.5819) (10.5761, -101.5961) (10.5993, -101.6008) knots 0 0 0 0 1 1 1 1
  line L158 (17.1126, -93.5277) -> (17.1258, -93.7171)
  line L159 (17.1258, -93.7171) -> (17.1302, -93.5281)
  spline S1977 degree 3 poles (17.1302, -93.5281) (17.1334, -93.3694) (17.1255, -93.305) (17.1059, -93.33) knots 0 0 0 0 1 1 1 1
  spline S1978 degree 3 poles (17.1059, -93.33) (17.1016, -93.3356) (17.1048, -93.4231) (17.1126, -93.5277) knots 0 0 0 0 1 1 1 1
  spline S1979 degree 3 poles (8.9329, -103.9744) (8.9437, -104.0007) (8.952, -104.0072) (8.9517, -103.9846) knots 0 0 0 0 1 1 1 1
  spline S1980 degree 3 poles (8.9517, -103.9846) (8.9493, -103.9648) (8.9788, -103.9386) (9.0178, -103.9287) knots 0 0 0 0 1 1 1 1
  spline S1981 degree 3 poles (9.0178, -103.9287) (9.0788, -103.9137) (9.076, -103.9115) (9.0054, -103.9102) knots 0 0 0 0 1 1 1 1
  spline S1982 degree 3 poles (9.0054, -103.9102) (8.9151, -103.9112) (8.908, -103.9146) (8.9329, -103.9744) knots 0 0 0 0 1 1 1 1
  spline S1983 degree 3 poles (10.9492, -101.6056) (11.0178, -101.6324) (11.0218, -101.6444) (10.9748, -101.6703) knots 0 0 0 0 1 1 1 1
  spline S1984 degree 3 poles (10.9748, -101.6703) (10.9283, -101.7012) (10.9289, -101.7061) (10.9861, -101.7016) knots 0 0 0 0 1 1 1 1
  spline S1985 degree 3 poles (10.9861, -101.7016) (11.0489, -101.7014) (11.0555, -101.6931) (11.0476, -101.6287) knots 0 0 0 0 1 1 1 1
  spline S1986 degree 3 poles (11.0476, -101.6287) (11.0396, -101.5643) (11.0264, -101.5584) (10.9521, -101.5675) knots 0 0 0 0 1 1 1 1
  spline S1987 degree 3 poles (10.9521, -101.5675) (10.8728, -101.5773) (10.8728, -101.5773) (10.9492, -101.6056) knots 0 0 0 0 1 1 1 1
  spline S1988 degree 3 poles (9.1496, -103.9377) (9.1551, -103.942) (9.1947, -103.9372) (9.2359, -103.9246) knots 0 0 0 0 1 1 1 1
  spline S1989 degree 3 poles (9.2359, -103.9246) (9.3046, -103.9111) (9.304, -103.9062) (9.2313, -103.9076) knots 0 0 0 0 1 1 1 1
  spline S1990 degree 3 poles (9.2313, -103.9076) (9.1586, -103.9089) (9.1273, -103.9203) (9.1496, -103.9377) knots 0 0 0 0 1 1 1 1
  spline S1991 degree 3 poles (17.104, -94.0717) (17.1054, -94.5339) (17.1254, -94.5943) (17.132, -94.1562) knots 0 0 0 0 1 1 1 1
  spline S1992 degree 3 poles (17.132, -94.1562) (17.136, -93.8415) (17.1283, -93.6967) (17.1078, -93.7344) knots 0 0 0 0 1 1 1 1
  spline S1993 degree 3 poles (17.1078, -93.7344) (17.1035, -93.74) (17.1019, -93.891) (17.104, -94.0717) knots 0 0 0 0 1 1 1 1
  spline S1994 degree 3 poles (10.2065, -102.6594) (10.2232, -102.6724) (10.2711, -102.674) (10.3123, -102.6615) knots 0 0 0 0 1 1 1 1
  spline S1995 degree 3 poles (10.3123, -102.6615) (10.3832, -102.6452) (10.3832, -102.6452) (10.3, -102.6429) knots 0 0 0 0 1 1 1 1
  spline S1996 degree 3 poles (10.3, -102.6429) (10.252, -102.6412) (10.2041, -102.6396) (10.1963, -102.638) knots 0 0 0 0 1 1 1 1
  spline S1997 degree 3 poles (10.1963, -102.638) (10.1864, -102.6392) (10.1898, -102.6463) (10.2065, -102.6594) knots 0 0 0 0 1 1 1 1
  spline S1998 degree 3 poles (10.5952, -102.202) (10.6007, -102.2063) (10.6404, -102.2015) (10.6815, -102.1889) knots 0 0 0 0 1 1 1 1
  spline S1999 degree 3 poles (10.6815, -102.1889) (10.7503, -102.1754) (10.7496, -102.1704) (10.6769, -102.1718) knots 0 0 0 0 1 1 1 1
  spline S2000 degree 3 poles (10.6769, -102.1718) (10.6042, -102.1732) (10.5729, -102.1846) (10.5952, -102.202) knots 0 0 0 0 1 1 1 1
  spline S2001 degree 3 poles (9.2958, -104.0027) (9.3465, -104.0065) (9.3778, -103.9951) (9.366, -103.9815) knots 0 0 0 0 1 1 1 1
  spline S2002 degree 3 poles (9.366, -103.9815) (9.3531, -103.9579) (9.3661, -103.9413) (9.4079, -103.9336) knots 0 0 0 0 1 1 1 1
  spline S2003 degree 3 poles (9.4079, -103.9336) (9.4618, -103.922) (9.4612, -103.917) (9.4086, -103.8983) knots 0 0 0 0 1 1 1 1
  spline S2004 degree 3 poles (9.4086, -103.8983) (9.3567, -103.8846) (9.3555, -103.8747) (9.3939, -103.8599) knots 0 0 0 0 1 1 1 1
  spline S2005 degree 3 poles (9.3939, -103.8599) (9.4273, -103.8458) (9.4289, -103.8381) (9.3985, -103.8368) knots 0 0 0 0 1 1 1 1
  spline S2006 degree 3 poles (9.3985, -103.8368) (9.3654, -103.8333) (9.3453, -103.8533) (9.3387, -103.9019) knots 0 0 0 0 1 1 1 1
  spline S2007 degree 3 poles (9.3387, -103.9019) (9.3293, -103.9483) (9.3048, -103.9739) (9.263, -103.9816) knots 0 0 0 0 1 1 1 1
  spline S2008 degree 3 poles (9.263, -103.9816) (9.2184, -103.987) (9.2317, -103.9929) (9.2958, -104.0027) knots 0 0 0 0 1 1 1 1
  spline S2009 degree 3 poles (7.2626, -106.5821) (7.2682, -106.5864) (7.3078, -106.5816) (7.3489, -106.569) knots 0 0 0 0 1 1 1 1
  spline S2010 degree 3 poles (7.3489, -106.569) (7.4177, -106.5555) (7.4171, -106.5506) (7.3443, -106.552) knots 0 0 0 0 1 1 1 1
  spline S2011 degree 3 poles (7.3443, -106.552) (7.2716, -106.5533) (7.2404, -106.5647) (7.2626, -106.5821) knots 0 0 0 0 1 1 1 1
  spline S2012 degree 3 poles (11.1503, -101.606) (11.1559, -101.6104) (11.1905, -101.6061) (11.2274, -101.5991) knots 0 0 0 0 1 1 1 1
  spline S2013 degree 3 poles (11.2274, -101.5991) (11.2664, -101.5893) (11.2822, -101.5748) (11.2655, -101.5617) knots 0 0 0 0 1 1 1 1
  spline S2014 degree 3 poles (11.2655, -101.5617) (11.2516, -101.5509) (11.217, -101.5551) (11.1885, -101.5687) knots 0 0 0 0 1 1 1 1
  spline S2015 degree 3 poles (11.1885, -101.5687) (11.1627, -101.5844) (11.1448, -101.6017) (11.1503, -101.606) knots 0 0 0 0 1 1 1 1
  spline S2016 degree 3 poles (16.5071, -94.7783) (16.521, -94.7891) (16.5529, -94.7827) (16.5765, -94.7698) knots 0 0 0 0 1 1 1 1
  spline S2017 degree 3 poles (16.5765, -94.7698) (16.6093, -94.7506) (16.6075, -94.7358) (16.571, -94.7252) knots 0 0 0 0 1 1 1 1
  spline S2018 degree 3 poles (16.571, -94.7252) (16.5163, -94.7093) (16.4682, -94.7479) (16.5071, -94.7783) knots 0 0 0 0 1 1 1 1
  spline S2019 degree 3 poles (15.3894, -96.2777) (15.4033, -96.2886) (15.4197, -96.279) (15.4222, -96.2586) knots 0 0 0 0 1 1 1 1
  spline S2020 degree 3 poles (15.4222, -96.2586) (15.4269, -96.2354) (15.4217, -96.2134) (15.4134, -96.2069) knots 0 0 0 0 1 1 1 1
  spline S2021 degree 3 poles (15.4134, -96.2069) (15.4078, -96.2026) (15.3936, -96.2093) (15.3805, -96.226) knots 0 0 0 0 1 1 1 1
  spline S2022 degree 3 poles (15.3805, -96.226) (15.3697, -96.2399) (15.3727, -96.2647) (15.3894, -96.2777) knots 0 0 0 0 1 1 1 1
  spline S2023 degree 3 poles (10.8734, -102.1955) (10.9482, -102.1913) (11.0188, -102.1927) (11.0287, -102.1915) knots 0 0 0 0 1 1 1 1
  spline S2024 degree 3 poles (11.0287, -102.1915) (11.0364, -102.193) (11.0429, -102.1847) (11.0411, -102.1698) knots 0 0 0 0 1 1 1 1
  spline S2025 degree 3 poles (11.0411, -102.1698) (11.0421, -102.1572) (10.9694, -102.1586) (10.8858, -102.1738) knots 0 0 0 0 1 1 1 1
  line L160 (10.8858, -102.1738) -> (10.7357, -102.1998)
  line L161 (10.7357, -102.1998) -> (10.8734, -102.1955)
  spline S2026 degree 3 poles (16.6696, -94.7709) (16.6752, -94.7752) (16.7148, -94.7704) (16.7559, -94.7578) knots 0 0 0 0 1 1 1 1
  spline S2027 degree 3 poles (16.7559, -94.7578) (16.8247, -94.7443) (16.8241, -94.7394) (16.7513, -94.7407) knots 0 0 0 0 1 1 1 1
  spline S2028 degree 3 poles (16.7513, -94.7407) (16.6786, -94.7421) (16.6474, -94.7535) (16.6696, -94.7709) knots 0 0 0 0 1 1 1 1
  spline S2029 degree 3 poles (7.4885, -106.5795) (7.494, -106.5838) (7.5336, -106.579) (7.5748, -106.5664) knots 0 0 0 0 1 1 1 1
  spline S2030 degree 3 poles (7.5748, -106.5664) (7.6435, -106.5529) (7.6429, -106.548) (7.5702, -106.5494) knots 0 0 0 0 1 1 1 1
  spline S2031 degree 3 poles (7.5702, -106.5494) (7.4975, -106.5507) (7.4662, -106.5621) (7.4885, -106.5795) knots 0 0 0 0 1 1 1 1
  spline S2032 degree 3 poles (9.5518, -103.9386) (9.5573, -103.9429) (9.597, -103.9381) (9.6381, -103.9255) knots 0 0 0 0 1 1 1 1
  spline S2033 degree 3 poles (9.6381, -103.9255) (9.7069, -103.912) (9.7063, -103.907) (9.6335, -103.9084) knots 0 0 0 0 1 1 1 1
  spline S2034 degree 3 poles (9.6335, -103.9084) (9.5608, -103.9098) (9.5295, -103.9212) (9.5518, -103.9386) knots 0 0 0 0 1 1 1 1
  spline S2035 degree 3 poles (10.0948, -103.2436) (10.1003, -103.2479) (10.1399, -103.2431) (10.1811, -103.2305) knots 0 0 0 0 1 1 1 1
  spline S2036 degree 3 poles (10.1811, -103.2305) (10.2498, -103.217) (10.2492, -103.2121) (10.1765, -103.2134) knots 0 0 0 0 1 1 1 1
  spline S2037 degree 3 poles (10.1765, -103.2134) (10.1038, -103.2148) (10.0725, -103.2262) (10.0948, -103.2436) knots 0 0 0 0 1 1 1 1
  spline S2038 degree 3 poles (9.7438, -103.8647) (9.7493, -103.8691) (9.789, -103.8642) (9.8301, -103.8516) knots 0 0 0 0 1 1 1 1
  spline S2039 degree 3 poles (9.8301, -103.8516) (9.8989, -103.8382) (9.8982, -103.8332) (9.8255, -103.8346) knots 0 0 0 0 1 1 1 1
  spline S2040 degree 3 poles (9.8255, -103.8346) (9.7528, -103.836) (9.7215, -103.8474) (9.7438, -103.8647) knots 0 0 0 0 1 1 1 1
  spline S2041 degree 3 poles (9.7777, -103.936) (9.7832, -103.9403) (9.8228, -103.9355) (9.864, -103.9229) knots 0 0 0 0 1 1 1 1
  spline S2042 degree 3 poles (9.864, -103.9229) (9.9327, -103.9094) (9.9321, -103.9044) (9.8594, -103.9058) knots 0 0 0 0 1 1 1 1
  spline S2043 degree 3 poles (9.8594, -103.9058) (9.7867, -103.9072) (9.7554, -103.9186) (9.7777, -103.936) knots 0 0 0 0 1 1 1 1
  spline S2044 degree 3 poles (10.3345, -103.2518) (10.3484, -103.2627) (10.3803, -103.2563) (10.4039, -103.2433) knots 0 0 0 0 1 1 1 1
  spline S2045 degree 3 poles (10.4039, -103.2433) (10.4367, -103.2242) (10.4349, -103.2094) (10.3984, -103.1988) knots 0 0 0 0 1 1 1 1
  spline S2046 degree 3 poles (10.3984, -103.1988) (10.3437, -103.1829) (10.2956, -103.2214) (10.3345, -103.2518) knots 0 0 0 0 1 1 1 1
  spline S2047 degree 3 poles (17.1071, -94.6292) (17.1128, -94.6964) (17.1026, -94.7152) (17.0459, -94.7247) knots 0 0 0 0 1 1 1 1
  spline S2048 degree 3 poles (17.0459, -94.7247) (16.9998, -94.7379) (16.9862, -94.7496) (17.0084, -94.767) knots 0 0 0 0 1 1 1 1
  spline S2049 degree 3 poles (17.0084, -94.767) (17.0251, -94.78) (17.0498, -94.777) (17.065, -94.7575) knots 0 0 0 0 1 1 1 1
  spline S2050 degree 3 poles (17.065, -94.7575) (17.0781, -94.7408) (17.0994, -94.7709) (17.1088, -94.8275) knots 0 0 0 0 1 1 1 1
  spline S2051 degree 3 poles (17.1088, -94.8275) (17.1211, -94.8864) (17.1295, -94.8527) (17.1304, -94.7369) knots 0 0 0 0 1 1 1 1
  spline S2052 degree 3 poles (17.1304, -94.7369) (17.1301, -94.5711) (17.1228, -94.5117) (17.1011, -94.5395) knots 0 0 0 0 1 1 1 1
  spline S2053 degree 3 poles (17.1011, -94.5395) (17.0989, -94.5422) (17.0988, -94.5825) (17.1071, -94.6292) knots 0 0 0 0 1 1 1 1
  spline S2054 degree 3 poles (9.9201, -103.8682) (9.9257, -103.8726) (9.9653, -103.8677) (10.0065, -103.8551) knots 0 0 0 0 1 1 1 1
  spline S2055 degree 3 poles (10.0065, -103.8551) (10.0752, -103.8416) (10.0746, -103.8367) (10.0019, -103.8381) knots 0 0 0 0 1 1 1 1
  spline S2056 degree 3 poles (10.0019, -103.8381) (9.9292, -103.8395) (9.8979, -103.8508) (9.9201, -103.8682) knots 0 0 0 0 1 1 1 1
  spline S2057 degree 3 poles (11.7673, -101.5956) (11.7812, -101.6065) (11.806, -101.6034) (11.819, -101.5868) knots 0 0 0 0 1 1 1 1
  spline S2058 degree 3 poles (11.819, -101.5868) (11.8299, -101.5729) (11.8203, -101.5564) (11.7999, -101.5539) knots 0 0 0 0 1 1 1 1
  spline S2059 degree 3 poles (11.7999, -101.5539) (11.7767, -101.5492) (11.7547, -101.5544) (11.7482, -101.5628) knots 0 0 0 0 1 1 1 1
  spline S2060 degree 3 poles (11.7482, -101.5628) (11.7439, -101.5683) (11.7506, -101.5826) (11.7673, -101.5956) knots 0 0 0 0 1 1 1 1
  spline S2061 degree 3 poles (10.497, -103.2445) (10.5026, -103.2488) (10.5422, -103.2439) (10.5833, -103.2314) knots 0 0 0 0 1 1 1 1
  spline S2062 degree 3 poles (10.5833, -103.2314) (10.6521, -103.2179) (10.6515, -103.2129) (10.5787, -103.2143) knots 0 0 0 0 1 1 1 1
  spline S2063 degree 3 poles (10.5787, -103.2143) (10.506, -103.2157) (10.4748, -103.2271) (10.497, -103.2445) knots 0 0 0 0 1 1 1 1
  spline S2064 degree 3 poles (10.0374, -104.0046) (10.043, -104.009) (10.0826, -104.0041) (10.1238, -103.9915) knots 0 0 0 0 1 1 1 1
  spline S2065 degree 3 poles (10.1238, -103.9915) (10.1925, -103.978) (10.1919, -103.9731) (10.1192, -103.9745) knots 0 0 0 0 1 1 1 1
  spline S2066 degree 3 poles (10.1192, -103.9745) (10.0464, -103.9759) (10.0152, -103.9872) (10.0374, -104.0046) knots 0 0 0 0 1 1 1 1
  line L162 (17.1114, -95.0534) -> (17.1341, -95.1562)
  line L163 (17.1341, -95.1562) -> (17.1312, -95.051)
  spline S2067 degree 3 poles (17.1312, -95.051) (17.1268, -94.9535) (17.1176, -94.9195) (17.1002, -94.9417) knots 0 0 0 0 1 1 1 1
  spline S2068 degree 3 poles (17.1002, -94.9417) (17.0959, -94.9473) (17.102, -94.9968) (17.1114, -95.0534) knots 0 0 0 0 1 1 1 1
  spline S2069 degree 3 poles (9.7513, -104.5198) (9.8036, -104.5159) (9.8504, -104.5076) (9.8569, -104.4993) knots 0 0 0 0 1 1 1 1
  spline S2070 degree 3 poles (9.8569, -104.4993) (9.8634, -104.4909) (9.8253, -104.4881) (9.773, -104.492) knots 0 0 0 0 1 1 1 1
  spline S2071 degree 3 poles (9.773, -104.492) (9.7207, -104.4959) (9.674, -104.5041) (9.6675, -104.5125) knots 0 0 0 0 1 1 1 1
  spline S2072 degree 3 poles (9.6675, -104.5125) (9.661, -104.5208) (9.699, -104.5237) (9.7513, -104.5198) knots 0 0 0 0 1 1 1 1
  spline S2073 degree 3 poles (13.562, -99.5506) (13.5676, -99.555) (13.6072, -99.5501) (13.6484, -99.5375) knots 0 0 0 0 1 1 1 1
  spline S2074 degree 3 poles (13.6484, -99.5375) (13.7171, -99.5241) (13.7165, -99.5191) (13.6437, -99.5205) knots 0 0 0 0 1 1 1 1
  spline S2075 degree 3 poles (13.6437, -99.5205) (13.571, -99.5219) (13.5398, -99.5333) (13.562, -99.5506) knots 0 0 0 0 1 1 1 1
  spline S2076 degree 3 poles (10.7229, -103.2419) (10.7284, -103.2462) (10.768, -103.2413) (10.8092, -103.2288) knots 0 0 0 0 1 1 1 1
  spline S2077 degree 3 poles (10.8092, -103.2288) (10.8779, -103.2153) (10.8773, -103.2103) (10.8046, -103.2117) knots 0 0 0 0 1 1 1 1
  spline S2078 degree 3 poles (10.8046, -103.2117) (10.7319, -103.2131) (10.7006, -103.2245) (10.7229, -103.2419) knots 0 0 0 0 1 1 1 1
  spline S2079 degree 3 poles (11.2368, -102.6585) (11.2507, -102.6694) (11.3086, -102.6698) (11.3674, -102.6576) knots 0 0 0 0 1 1 1 1
  line L164 (11.3674, -102.6576) -> (11.468, -102.6377)
  line L165 (11.468, -102.6377) -> (11.3551, -102.639)
  spline S2080 degree 3 poles (11.3551, -102.639) (11.2923, -102.6391) (11.2344, -102.6387) (11.2267, -102.6371) knots 0 0 0 0 1 1 1 1
  spline S2081 degree 3 poles (11.2267, -102.6371) (11.2168, -102.6384) (11.2201, -102.6455) (11.2368, -102.6585) knots 0 0 0 0 1 1 1 1
  spline S2082 degree 3 poles (10.331, -103.8982) (10.339, -103.9223) (10.325, -103.9517) (10.2993, -103.9674) knots 0 0 0 0 1 1 1 1
  spline S2083 degree 3 poles (10.2993, -103.9674) (10.2735, -103.9832) (10.2754, -103.998) (10.3118, -104.0086) knots 0 0 0 0 1 1 1 1
  spline S2084 degree 3 poles (10.3118, -104.0086) (10.3406, -104.0176) (10.3719, -104.0063) (10.3787, -103.9803) knots 0 0 0 0 1 1 1 1
  spline S2085 degree 3 poles (10.3787, -103.9803) (10.3884, -103.9565) (10.4178, -103.9303) (10.4448, -103.9244) knots 0 0 0 0 1 1 1 1
  spline S2086 degree 3 poles (10.4448, -103.9244) (10.4788, -103.9152) (10.476, -103.9131) (10.4386, -103.9151) knots 0 0 0 0 1 1 1 1
  spline S2087 degree 3 poles (10.4386, -103.9151) (10.3362, -103.9202) (10.3307, -103.8756) (10.4291, -103.8585) knots 0 0 0 0 1 1 1 1
  spline S2088 degree 3 poles (10.4291, -103.8585) (10.5297, -103.8386) (10.5297, -103.8386) (10.4354, -103.8276) knots 0 0 0 0 1 1 1 1
  spline S2089 degree 3 poles (10.4354, -103.8276) (10.3361, -103.8171) (10.3082, -103.8356) (10.331, -103.8982) knots 0 0 0 0 1 1 1 1
  spline S2090 degree 3 poles (17.103, -95.8034) (17.1053, -96.1499) (17.1117, -96.4683) (17.1194, -96.5101) knots 0 0 0 0 1 1 1 1
  spline S2091 degree 3 poles (17.1194, -96.5101) (17.127, -96.5519) (17.1303, -96.4962) (17.1317, -96.3855) knots 0 0 0 0 1 1 1 1
  spline S2092 degree 3 poles (17.1317, -96.3855) (17.1351, -95.2465) (17.1336, -95.111) (17.1078, -95.167) knots 0 0 0 0 1 1 1 1
  spline S2093 degree 3 poles (17.1078, -95.167) (17.1034, -95.1725) (17.1034, -95.459) (17.103, -95.8034) knots 0 0 0 0 1 1 1 1
  spline S2094 degree 3 poles (9.9001, -104.5241) (9.9057, -104.5285) (9.9453, -104.5236) (9.9865, -104.511) knots 0 0 0 0 1 1 1 1